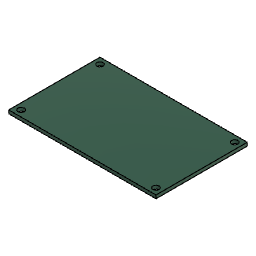
AssemblyNewMainBoard v2 (Autodesk Fusion 360 archive; units mm, degrees)
design "MainBoardMotorDrivers"
Autodesk Fusion 360 part; units mm, degrees
sketch "Sketch1" plane through (0, 0, 0) normal (0, 0, 1) x (1, 0, 0)
  line L0 (-35.5, 22) -> (35.5, 22)
  line L1 (35.5, 22) -> (35.5, -22)
  line L2 (35.5, -22) -> (-35.5, -22)
  line L3 (-35.5, -22) -> (-35.5, 22)
  line L4 (0, 0) -> (-35.5, 0) construction
  line L5 (0, 0) -> (0, 22) construction
  circle A0 centre (-32.5, 19) radius 1.5
  circle A1 centre (32.5, 19) radius 1.5
  circle A2 centre (-32.5, -19) radius 1.5
  circle A3 centre (32.5, -19) radius 1.5
  point P0 (-35.5, 0)
  point P1 (0, 22)
  dimension "d1" = 71
  dimension "d2" = 44
  dimension "d3" = 3
  dimension "d4" = 3
  dimension "d5" = 3
  dimension "d8" = 65
  dimension "d9" = -38
  constraint horizontal L0
  constraint vertical L1
  constraint horizontal L2
  constraint vertical L3
  constraint midpoint L3 P0
  constraint midpoint L0 P1
  constraint coincident L4.start L5.start
  constraint coincident P0 L4.end
  constraint coincident P1 L5.end
  constraint vertical L5
  constraint horizontal L4
  measures "d1" distance of L0.start L0.end
  measures "d2" distance of L0.start L2.end
  measures "d3" diameter of A0
  measures "d4" distance of L3 A0.centre
  measures "d5" distance of L0 A0.centre
extrude "Extrude1" add sketch "Sketch1" along normal blind 1.591
